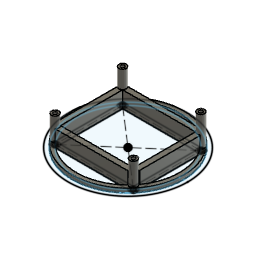
Sat Stand 3 (Autodesk Fusion 360 design; units mm, degrees)
Autodesk Fusion 360 part; units mm, degrees
sketch "Sketch1" plane through (0, 0, 0) normal (0, 1, 0) x (1, 0, 0)
  circle A0 centre (0, 0) radius 44
  line L0 (28.875, 24.875) -> (-28.875, 24.875) construction
  line L1 (-28.875, 24.875) -> (-28.875, -24.875) construction
  line L2 (-28.875, -24.875) -> (28.875, -24.875) construction
  line L3 (28.875, -24.875) -> (28.875, 24.875) construction
  line L4 (28.875, 24.875) -> (-28.875, -24.875) construction
  line L5 (-28.875, 24.875) -> (28.875, -24.875) construction
  circle A1 centre (-28.875, 24.875) radius 1.375
  circle A2 centre (-28.875, 24.875) radius 2.75
  circle A3 centre (-28.875, -24.875) radius 1.375
  circle A4 centre (-28.875, -24.875) radius 2.75
  circle A5 centre (28.875, 24.875) radius 1.375
  circle A6 centre (28.875, 24.875) radius 2.75
  circle A7 centre (28.875, -24.875) radius 1.375
  circle A8 centre (28.875, -24.875) radius 2.75
  circle A9 centre (0, 0) radius 40.9963
  circle A10 centre (0, 0) radius 37.9963
  line L6 (30.875, 26.875) -> (-30.875, 26.875)
  line L7 (-30.875, 26.875) -> (-30.875, -26.875)
  line L8 (-30.875, -26.875) -> (30.875, -26.875)
  line L9 (30.875, -26.875) -> (30.875, 26.875)
  line L10 (26.875, 22.875) -> (-26.875, 22.875)
  line L11 (-26.875, 22.875) -> (-26.875, -22.875)
  line L12 (-26.875, -22.875) -> (26.875, -22.875)
  line L13 (26.875, -22.875) -> (26.875, 22.875)
  dimension "d1" = 88
  dimension "d2" = 57.75
  dimension "d3" = 49.75
  dimension "d4" = 2.75
  dimension "d5" = 5.5
  dimension "d6" = 2.75
  dimension "d7" = 5.5
  dimension "d8" = 2.75
  dimension "d9" = 5.5
  dimension "d10" = 2.75
  dimension "d11" = 5.5
  dimension "d30" = -3
  dimension "d41" = 2
  dimension "d42" = -2
  constraint coincident A0.centre A9.centre
  constraint horizontal L0
  constraint perpendicular L0 L1
  constraint parallel L0 L2
  constraint parallel L1 L3
  constraint coincident L4 A0.centre
  constraint coincident L5 A0.centre
  constraint coincident L0.end L1.start
  constraint concentric A1 A2
  constraint coincident L1.end L2.start
  constraint concentric A3 A4
  constraint coincident L0.start L3.end
  constraint concentric A5 A6
  constraint coincident L2.end L3.start
  constraint concentric A7 A8
  constraint concentric A0 A9
  measures "d1" diameter of A0
  measures "d2" distance of L1.end L2.end
  measures "d3" distance of L0.end L1.end
  measures "d4" diameter of A1
  measures "d5" diameter of A2
  measures "d6" diameter of A3
  measures "d7" diameter of A4
  measures "d8" diameter of A5
  measures "d9" diameter of A6
  measures "d10" diameter of A7
  measures "d11" diameter of A8
extrude "Extrude7" add sketch "Sketch1" along normal blind 3 contours A2 A10 L6 | A2 A10 L7 | A2 L6 L7 | A6 A10 L6 | A4 A10 L7 | A6 A10 L9 | A6 L6 L9 | A4 L7 L8 | A4 A10 L8 | A8 A10 L9 | A8 A10 L8 | A8 L8 L9 | A9
extrude "Extrude9" add sketch "Sketch1" along normal blind 20 contours A3 A4 A10 L7 L8 | A3 A4 A10 | A4 L7 | A4 L8 | A7 A8 A10 | A7 A8 A10 L8 L9 | A8 L9 | A8 L8
extrude "Extrude10" add sketch "Sketch1" along normal blind 25 contours A1 A2 A10 | A1 A2 A10 L6 L7 | A2 L6 | A2 L7 | A5 A6 A10 | A5 A6 A10 L6 L9 | A6 L6 | A6 L9
extrude "Extrude11" add sketch "Sketch1" along normal blind 12 contours A2 A4 A6 A8 A10 L6 L7 L8 L9
extrude "Extrude12" add sketch "Sketch1" along normal blind 15 contours A1 A10 | A1 A10 | A5 A10 | A5 A10 | A3 A10 | A3 A10 | A7 A10 | A7 A10
equation "d2 = 55 mm + 2.75 mm"
equation "d3 = 48 mm + 1.75 mm"
named bodies: "sat stand 3"
